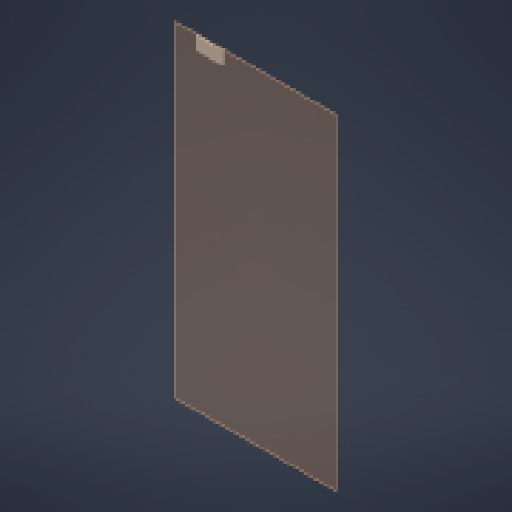
# Autodesk Inventor part: 0110_v2
Saved by Autodesk Inventor 2024 (Build 280153000, 153)
## iProperties
Created: 2023-05-19
Part Number: 0110_v2
Material: Genérico
Document SubType Name: Sheet Metal
Designer: javie
Density: 1 g/cm^3
Sheet Metal Rule: Por defecto_mm
Appearance: Valor por defecto
Author: javie
Autodesk Inventor part; units mm, degrees
ref_plane "YZ Plane" through (0, 0, 0) normal (1, 0, 0) x (0, 1, 0)
ref_plane "XZ Plane" through (0, 0, 0) normal (0, 1, 0) x (-1, 0, 0)
ref_plane "XY Plane" through (0, 0, 0) normal (0, 0, 1) x (1, 0, 0)
ref_plane "Plano de trabajo1" through (0, 0, 0) normal (0, 0, 1) x (1, 0, 0)
sketch "Boceto1" plane through (0, 0, 0) normal (0, 0, 1) x (1, 0, 0)
  line L0 (-164.2, 333) -> (-44.2, 333)
  line L1 (-44.2, 333) -> (-44.2, 363)
  line L2 (-44.2, 363) -> (-164.2, 363)
  line L3 (-164.2, 363) -> (-164.2, 333)
  line L4 (-104.2, 363) -> (-104.2, 333)
  line L5 (-74.2, 363) -> (-74.2, 333)
  line L6 (-134.2, 363) -> (-134.2, 333)
  point P0 (0, 0)
  dimension "d0" = 120
  dimension "d1" = 30
  dimension "d2" = 30
  dimension "d3" = 30
  constraints: 14 end point, 4 point on line, 3 perpendicular, 2 midpoint, 2 parallel, 1 horizontal
  measures "d0" distance of L2.end L1.end
  measures "d1" distance of L1.end L0.end
  measures "d2" distance between parallel lines of L3 L6
  measures "d3" distance between parallel lines of L1 L5
extrude "Extrusión1" add sketch "Boceto1" against normal blind 2 contours L6 L2 L4 L0 | L4 L2 L5 L0
equation "\"Radio_pliegue\" = Grosor"
equation "\"Anchura_desahogo_plegado\" = Grosor"
equation "\"Profundidad_desahogo_plegado\" = 0.5 * Grosor"
equation "\"Tamaño_destalonado\" = 4 * Grosor"
equation "\"Remanente_mínimo\" = 2 * Grosor"
equation "\"Radiodetransición\" = Radio_pliegue"
equation "\"Tamaño_de_radio_de_Jacobi\" = Radio_pliegue"
equation "\"TamañoSeparación\" = Grosor"
equation "\"Grosor\" = 0.5"
